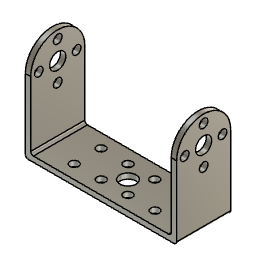
双轴舵机支架2 v2 (Autodesk Fusion 360 design; units mm, degrees)
Autodesk Fusion 360 part; units mm, degrees
note: some values were not read from the file. Set by a fixed rule: which sketch regions a step uses.
sketch "草图1" plane through (0, 0, 0) normal (0, 0, 1) x (1, 0, 0)
  line L0 (0, 0) -> (56, 0)
  line L1 (56, 0) -> (56, 20)
  line L2 (56, 20) -> (0, 20)
  line L3 (0, 20) -> (0, 0)
  dimension "d1" = 56
  dimension "d2" = 20
  constraint horizontal L0
  constraint vertical L1
  constraint horizontal L2
  constraint vertical L3
  constraint coincident L0.start L3.end
  measures "d1" distance of L0.start L0.end
  measures "d2" distance of L0.start L2.end
extrude "拉伸1" add sketch "草图1" along normal blind 2 makes body 1
sketch "草图2" plane through (0, 0, 2) normal (0, 0, 1) x (-1, 0, 0)
  line L0 (0, -20) -> (0, 0)
  line L1 (0, 0) -> (-56, 0)
  line L2 (-56, 0) -> (-56, -20)
  line L3 (-56, -20) -> (0, -20)
  line L4 (-10, -10) -> (-50.5346, -10)
  line L5 (-28, -17) -> (-28, -4)
  circle A0 centre (-28, -10) radius 3
  circle A1 centre (-28, -10) radius 7 construction
  line L6 (-28, -10) -> (-35.6485, -17.6485) construction
  circle A2 centre (-32.9497, -14.9497) radius 1.6
  circle A3 centre (-23.0503, -14.9497) radius 1.6
  circle A4 centre (-23.0503, -5.0503) radius 1.6
  circle A5 centre (-32.9497, -5.0503) radius 1.6
  circle A6 centre (-42.9497, -14.9497) radius 1.6
  circle A7 centre (-42.9497, -5.0503) radius 1.6
  circle A8 centre (-13.0503, -14.9497) radius 1.6
  circle A9 centre (-13.0503, -5.0503) radius 1.6
  dimension "d5" = 6
  dimension "d6" = 14
  dimension "d7" = 45
  dimension "d8" = 3.2
  dimension "d10" = 360
  dimension "d13" = -10
  dimension "d14" = 3
  constraint horizontal L4
  constraint perpendicular L4 L5
  constraint symmetric L0 L2 L5
  constraint symmetric L1 L3 L4
  constraint coincident L5 A0.centre
  constraint coincident L4 A0.centre
  constraint concentric A0 A1
  constraint coincident A0.centre A1.centre
  constraint coincident A1 A2.centre
  constraint coincident L6 A2.centre
  constraint symmetric L4 A6 A7
  constraint symmetric L5 A6 A8
  constraint symmetric L5 A7 A9
  measures "d5" diameter of A0
  measures "d6" diameter of A1
  measures "d7" angle of L4 L6
  measures "d8" diameter of A2
extrude "拉伸2" cut sketch "草图2" against normal blind 2 contours L4 L5 A0 | L4 L5 A0 | L4 L5 A0 | L4 L5 A0 | A2 | A3 | A4 | A5 | A6 | A7 | A8 | A9 bodies 1
sketch "草图3" plane through (0, 0, 2) normal (0, 0, 1) x (-1, 0, 0)
  circle A0 centre (-42.9497, -14.9497) radius 1.6
  circle A1 centre (-23.0503, -14.9497) radius 1.6
  circle A2 centre (-13.0503, -5.0503) radius 1.6
  circle A3 centre (-32.9497, -14.9497) radius 1.6
  circle A4 centre (-42.9497, -5.0503) radius 1.6
  circle A5 centre (-28, -10) radius 3
  circle A6 centre (-13.0503, -14.9497) radius 1.6
  circle A7 centre (-23.0503, -5.0503) radius 1.6
  circle A8 centre (-32.9497, -5.0503) radius 1.6
  line L0 (0, -20) -> (0, 0)
  line L1 (0, 0) -> (-56, 0)
  line L2 (-56, 0) -> (-56, -20)
  line L3 (-56, -20) -> (0, -20)
  line L4 (0, 0) -> (-2, 0)
  line L5 (-2, 0) -> (-2, -20)
  line L6 (-2, -20) -> (0, -20)
  line L7 (0, -20) -> (0, 0)
  line L8 (-56, 0) -> (-54, 0)
  line L9 (-54, 0) -> (-54, -20)
  line L10 (-54, -20) -> (-56, -20)
  line L11 (-56, -20) -> (-56, 0)
  dimension "d17" = 2
  dimension "d18" = 2
  constraint horizontal L4
  constraint vertical L5
  constraint horizontal L6
  constraint vertical L7
  constraint coincident L3 L5.end
  constraint coincident L0.end L1.start
  constraint horizontal L8
  constraint vertical L9
  constraint horizontal L10
  constraint vertical L11
  constraint coincident L3 L9.end
  constraint coincident L1.end L2.start
  measures "d17" distance of L5.end L0.start
  measures "d18" distance of L9.end L2.end
extrude "拉伸3" add sketch "草图3" along normal blind 35 contours L0 L1 L3 L4 L5 L6 L7 | L1 L2 L3 L8 L9 L10 L11 bodies 1
fillet "圆角1" radius 1 4 edges at (56, 10, 0) (54, 10, 2) (2, 10, 2) (0, 10, 0) on bodies 1
sketch "草图4" plane through (56, 0, 0) normal (1, 0, 0) x (0, 1, 0)
  line L0 (0, 1) -> (20, 1)
  line L1 (20, 1) -> (20, 37)
  line L2 (20, 37) -> (0, 37)
  line L3 (0, 37) -> (0, 1)
  circle A0 centre (10, 27) radius 7 construction
  line L4 (0, 27) -> (0, 37)
  line L5 (20, 37) -> (20, 27)
  arc A1 (20, 26.9983) -> (0, 27) centre (10, 27) ccw
  line L6 (10, 27) -> (19, 27) construction
  circle A2 centre (17, 27) radius 1.6
  circle A3 centre (10, 34) radius 1.6
  circle A4 centre (3, 27) radius 1.6
  circle A5 centre (10, 20) radius 1.6
  circle A6 centre (10, 27) radius 3
  dimension "d23" = 14
  dimension "d24" = 27
  dimension "d25" = 20
  dimension "d26" = 3.2
  dimension "d28" = 360
  dimension "d29" = 6
  constraint concentric A0 A1
  constraint coincident L3 L4.start
  constraint coincident L2.end L3.start
  constraint perpendicular L2 L4
  constraint coincident L1.end L2.start
  constraint coincident L5.end A1
  constraint coincident L1 L5.end
  constraint coincident L1 A1.start
  constraint coincident A0.centre A1.centre
  constraint perpendicular L4 L6
  constraint coincident A0 A2.centre
  constraint coincident L6 A2.centre
  measures "d23" diameter of A0
  measures "d24" vertical distance of origin A0.centre
  measures "d25" diameter of A1
  measures "d26" diameter of A2
  measures "d29" diameter of A6
extrude "拉伸4" cut sketch "草图4" against normal blind 56 contours L2 L3 L4 A1 | L1 L2 L5 A1 | A2 | A3 | A4 | A5 | A6 bodies 1
copy_body "实体->零部件1" bodies 1 removing the originals makes body 2 in component "Component'"
component "Component'" placed x (1, 0, 0) y (0, 1, 0) z (0, 0, 1) at (0, 0, 0)
